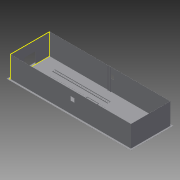
# Autodesk Inventor part: NIST_NRC_Drawing
Saved by Autodesk Inventor 2013 SP2 (Build 170200200, 200)
## iProperties
Created: 2014-01-14
Part Number: NIST_NRC_Drawing
Material: Generic
Document SubType Name: Modeling
Designer: mcgratta
Density: 1 g/cm^3
Author: mcgratta
Autodesk Inventor part; units mm, degrees
ref_plane "YZ Plane" through (0, 0, 0) normal (1, 0, 0) x (0, 1, 0)
ref_plane "XZ Plane" through (0, 0, 0) normal (0, 1, 0) x (-1, 0, 0)
sketch "Sketch1" plane through (0, 0, 0) normal (0, 1, 0) x (-1, 0, 0)
  line L0 (300, 300) -> (-21960, 300)
  line L1 (-21960, 300) -> (-21960, -7340)
  line L2 (-21960, -7340) -> (300, -7340)
  line L3 (300, -7340) -> (300, 300)
  point P0 (0, 0)
  dimension "d0" = 300
  dimension "d1" = 22260
  dimension "d2" = 300
  dimension "d3" = 7640
  constraints: 8 end point, 2 parallel, 1 horizontal, 1 perpendicular
  measures "d0" distance from line of L3 point (0, 0)
  measures "d1" distance between parallel lines of L1 L3
  measures "d2" distance from line of L0 point (0, 0)
  measures "d3" distance between parallel lines of L2 L0
extrude "Extrusion2" add sketch "Sketch1" against normal blind 10
sketch "Sketch4" plane through (0, 0, 0) normal (0, 1, 0) x (1, 0, 0)
  line L0 (0, 0) -> (21700, 0)
  line L1 (21700, 0) -> (21700, 20)
  line L2 (21700, 20) -> (0, 20)
  line L3 (0, 20) -> (0, 0)
  dimension "d28" = 20
  dimension "d30" = 21700
  constraints: 8 end point, 2 parallel, 1 horizontal, 1 perpendicular
  measures "d28" distance between parallel lines of L0 L2
  measures "d30" distance between parallel lines of L1 L3
extrude "Extrusion4" add sketch "Sketch4" along normal blind 3820
sketch "Sketch5" plane through (0, 0, 0) normal (0, 1, 0) x (1, 0, 0)
  line L0 (0, 20) -> (21700, 20) projected
  line L1 (0, 20) -> (20, 20)
  line L2 (20, 20) -> (20, 7060)
  line L3 (20, 7060) -> (0, 7060)
  line L4 (0, 7060) -> (0, 20)
  dimension "d33" = 20
  dimension "d35" = 7040
  constraints: 8 end point, 2 parallel, 1 horizontal, 1 perpendicular
  measures "d33" distance between parallel lines of L2 L4
  measures "d35" distance between parallel lines of L3 L0
extrude "Extrusion5" add sketch "Sketch5" along normal blind 3820
sketch "Sketch6" plane through (0, 0, 0) normal (0, 1, 0) x (1, 0, 0)
  line L0 (0, 7060) -> (21700, 7060)
  line L1 (21700, 7060) -> (21700, 7080)
  line L2 (21700, 7080) -> (0, 7080)
  line L3 (0, 7080) -> (0, 7060)
  dimension "d38" = 20
  dimension "d40" = 21700
  constraints: 8 end point, 2 parallel, 1 horizontal, 1 perpendicular
  measures "d38" distance between parallel lines of L0 L2
  measures "d40" distance between parallel lines of L1 L3
extrude "Extrusion6" add sketch "Sketch6" along normal blind 3820
sketch "Sketch7" plane through (0, 0, 0) normal (0, 1, 0) x (1, 0, 0)
  line L0 (0, 20) -> (21700, 20) projected
  line L1 (21700, 20) -> (21680, 20)
  line L2 (21680, 20) -> (21680, 7060)
  line L3 (21680, 7060) -> (21700, 7060)
  line L4 (21700, 7060) -> (21700, 20)
  point P0 (20, 20)
  dimension "d43" = 20
  dimension "d45" = 7040
  constraints: 8 end point, 2 parallel, 1 horizontal, 1 perpendicular
  measures "d43" distance between parallel lines of L4 L2
  measures "d45" distance between parallel lines of L3 L0
extrude "Extrusion7" add sketch "Sketch7" along normal blind 3820
sketch "Sketch10" plane through (20, 0, -20) normal (1, 0, 0) x (0, 0, -1)
  line L0 (7040, 0) -> (0, 0) projected
  line L1 (7040, 0) -> (7040, 3820) projected
  line L2 (0, 3820) -> (7040, 3820) projected
  line L3 (0, 0) -> (0, 3820) projected
  point P0 (-20, 0)
sketch "Sketch11" plane through (0, 0, 0) normal (-1, 0, 0) x (0, 0, 1)
  line L0 (0, 0) -> (-7080, 0) projected
  line L1 (-7080, 0) -> (-7080, 3820) projected
  line L2 (-4560, 0) -> (-2560, 0)
  line L3 (-2560, 0) -> (-2560, 2000)
  line L4 (-2560, 2000) -> (-4560, 2000)
  line L5 (-4560, 2000) -> (-4560, 0)
  dimension "d73" = 2000
  dimension "d75" = 2000
  dimension "d76" = 2520
  constraints: 8 end point, 2 parallel, 1 horizontal, 1 perpendicular, 1 point on line
  measures "d73" distance between parallel lines of L3 L5
  measures "d75" distance of L2.end L3.end
  measures "d76" distance between parallel lines of L1 L5
extrude "Extrusion10" cut sketch "Sketch11" along normal mid plane 40
sketch "Sketch12" plane through (0, 0, 0) normal (0, 0, 1) x (1, 0, 0)
  line L0 (21700, 0) -> (0, 0) projected
  line L1 (0, 0) -> (0, 3820) projected
  line L2 (10870, 2050) -> (11570, 2050)
  line L3 (11570, 2050) -> (11570, 2750)
  line L4 (11570, 2750) -> (10870, 2750)
  line L5 (10870, 2750) -> (10870, 2050)
  line L6 (10870, 2050) -> (11570, 2750) construction
  line L7 (11570, 2050) -> (10870, 2750) construction
  point P0 (11220, 2400)
  dimension "d79" = 2400
  dimension "d80" = 700
  dimension "d81" = 700
  dimension "d82" = 11220
  constraints: 12 end point, 2 midpoint, 2 parallel, 1 horizontal, 1 perpendicular
  measures "d79" distance from line of L0 point (11220, 2400)
  measures "d80" distance of L2.start L2.end
  measures "d81" distance of L4.end L2.start
  measures "d82" distance from line of L1 point (11220, 2400)
extrude "Extrusion11" cut sketch "Sketch12" along normal mid plane 40
sketch "Sketch13" plane through (21700, 0, -7080) normal (0, 0, -1) x (-1, 0, 0)
  line L0 (21700, 0) -> (0, 0) projected
  line L1 (21700, 0) -> (21700, 3820) projected
  line L2 (10130, 2050) -> (10830, 2050)
  line L3 (10830, 2050) -> (10830, 2750)
  line L4 (10830, 2750) -> (10130, 2750)
  line L5 (10130, 2750) -> (10130, 2050)
  line L6 (10130, 2050) -> (10830, 2750) construction
  line L7 (10830, 2050) -> (10130, 2750) construction
  point P0 (10480, 2400)
  dimension "d85" = 11220
  dimension "d86" = 2400
  dimension "d87" = 700
  dimension "d88" = 700
  constraints: 12 end point, 2 midpoint, 2 parallel, 1 horizontal, 1 perpendicular
  measures "d85" distance from line of L1 point (10480, 2400)
  measures "d86" distance from line of L0 point (10480, 2400)
  measures "d87" distance of L2.start L2.end
  measures "d88" distance of L4.end L2.start
extrude "Extrusion12" cut sketch "Sketch13" against normal blind 40
sketch "Sketch14" plane through (0, 0, 0) normal (0, 1, 0) x (1, 0, 0)
  line L0 (21680, 7060) -> (20, 7060) projected
  line L1 (20, 7060) -> (20, 4560) projected
  line L2 (11850, 3040) -> (9850, 3040)
  line L3 (9850, 3040) -> (9850, 4040)
  line L4 (9850, 4040) -> (11850, 4040)
  line L5 (11850, 4040) -> (11850, 3040)
  line L6 (11850, 3040) -> (9850, 4040) construction
  line L7 (9850, 3040) -> (11850, 4040) construction
  line L8 (9840, 4050) -> (11860, 4050)
  line L9 (11860, 4050) -> (11860, 3030)
  line L10 (11860, 3030) -> (9840, 3030)
  line L11 (9840, 3030) -> (9840, 4050)
  point P0 (10850, 3540)
  point P1 (0, 7060)
  dimension "d91" = 10830
  dimension "d92" = 3520
  dimension "d93" = 2000
  dimension "d94" = 1000
  dimension "d95" = 10
  dimension "d96" = 10
  dimension "d97" = 10
  dimension "d98" = 10
  constraints: 20 end point, 4 parallel, 2 horizontal, 2 midpoint, 2 perpendicular
  measures "d91" distance from line of L1 point (10850, 3540)
  measures "d92" distance from line of L0 point (10850, 3540)
  measures "d93" distance of L2.start L2.end
  measures "d94" distance of L2.end L3.end
  measures "d95" distance between parallel lines of L4 L8
  measures "d96" distance between parallel lines of L3 L11
  measures "d97" distance between parallel lines of L2 L10
  measures "d98" distance between parallel lines of L5 L9
extrude "Extrusion13" add sketch "Sketch14" along normal blind 100
ref_plane "Work Plane1" through (15850, 0, -7060) normal (-1, 0, 0) x (0, 0, 1)
sketch "Sketch16" plane through (15850, 0, -7060) normal (-1, 0, 0) x (0, 0, 1)
  circle A0 centre (4840, 3200) radius 10
  line L0 (-280, 0) -> (7360, 0) projected
  line L1 (7040, 0) -> (7040, 3820) projected
  line L2 (4890, 3210) -> (5340, 3210)
  line L3 (5340, 3210) -> (5340, 3200)
  line L4 (5340, 3200) -> (4890, 3200)
  line L5 (4890, 3200) -> (4890, 3210)
  line L6 (4890, 3210) -> (4900, 3210)
  line L7 (4900, 3210) -> (4900, 3310)
  line L8 (4900, 3310) -> (4890, 3310)
  line L9 (4890, 3310) -> (4890, 3210)
  line L10 (5340, 3210) -> (5330, 3210)
  line L11 (5330, 3210) -> (5330, 3310)
  line L12 (5330, 3310) -> (5340, 3310)
  line L13 (5340, 3310) -> (5340, 3210)
  circle A1 centre (5015, 3220) radius 10
  circle A2 centre (5115, 3220) radius 10
  circle A3 centre (5215, 3220) radius 10
  circle A4 centre (5690, 2700) radius 10
  circle A5 centre (6440, 2200) radius 10
  circle A6 centre (6540, 2200) radius 10
  point P0 (7060, 0)
  dimension "d102" = 3200
  dimension "d103" = 2200
  dimension "d104" = 20
  dimension "d105" = 10
  dimension "d106" = 50
  dimension "d107" = 0
  dimension "d108" = 450
  dimension "d109" = 10
  dimension "d110" = 100
  dimension "d111" = 10
  dimension "d112" = 100
  dimension "d113" = 20
  dimension "d114" = 20
  dimension "d115" = 20
  dimension "d116" = 10
  dimension "d117" = 10
  dimension "d118" = 10
  dimension "d119" = 225
  dimension "d120" = 100
  dimension "d121" = 100
  dimension "d122" = 2700
  dimension "d123" = 1350
  dimension "d124" = 20
  dimension "d125" = 2200
  dimension "d126" = 2200
  dimension "d127" = 600
  dimension "d128" = 500
  dimension "d129" = 20
  dimension "d130" = 20
  constraints: 24 end point, 7 centre point, 6 parallel, 3 horizontal, 3 perpendicular
  measures "d102" distance from line of L0 A0.centre
  measures "d103" distance from line of L1 A0.centre
  measures "d104" diameter of A0
  measures "d105" distance between parallel lines of L4 L2
  measures "d106" horizontal distance of L2.start A0.centre
  measures "d107" distance from line of A0.centre L4
  measures "d108" distance of L3.end L4.end
  measures "d109" distance between parallel lines of L7 L9
  measures "d110" distance of L8.end L2.start
  measures "d111" distance between parallel lines of L13 L11
  measures "d112" vertical distance of L10.end L12.end
  measures "d113" diameter of A1
  measures "d114" diameter of A2
  measures "d115" diameter of A3
  measures "d116" distance from line of L2 A1.centre
  measures "d117" distance from line of L2 A2.centre
  measures "d118" distance from line of L2 A3.centre
  measures "d119" distance from line of L9 A2.centre
  measures "d120" distance of A1.centre A2.centre
  measures "d121" distance of A2.centre A3.centre
  measures "d122" distance from line of L0 A4.centre
  measures "d123" distance from line of L1 A4.centre
  measures "d124" diameter of A4
  measures "d125" distance from line of L0 A5.centre
  measures "d126" distance from line of L0 A6.centre
  measures "d127" distance from line of L1 A5.centre
  measures "d128" distance from line of L1 A6.centre
  measures "d129" diameter of A5
  measures "d130" diameter of A6
extrude "Extrusion14" add sketch "Sketch16" along normal blind 10000
sketch "Sketch17" plane through (0, 0, 0) normal (0, 1, 0) x (1, 0, 0)
  line L0 (21680, 7060) -> (20, 7060) projected
  line L1 (20, 7060) -> (20, 4560) projected
  line L2 (10600, 7010) -> (11050, 7010)
  line L3 (11050, 7010) -> (11050, 7000)
  line L4 (11050, 7000) -> (10600, 7000)
  line L5 (10600, 7000) -> (10600, 7010)
  line L6 (10600, 7000) -> (10610, 7000)
  line L7 (10610, 7000) -> (10610, 6900)
  line L8 (10610, 6900) -> (10600, 6900)
  line L9 (10600, 6900) -> (10600, 7000)
  line L10 (11050, 7000) -> (11040, 7000)
  line L11 (11040, 7000) -> (11040, 6900)
  line L12 (11040, 6900) -> (11050, 6900)
  line L13 (11050, 6900) -> (11050, 7000)
  dimension "d133" = 450
  dimension "d135" = 10
  dimension "d136" = 10
  dimension "d137" = 10
  dimension "d139" = 100
  dimension "d140" = 100
  dimension "d141" = 50
  dimension "d142" = 10580
  constraints: 24 end point, 6 parallel, 3 horizontal, 3 perpendicular
  measures "d133" distance of L2.start L2.end
  measures "d135" distance between parallel lines of L4 L2
  measures "d136" distance between parallel lines of L9 L7
  measures "d137" distance between parallel lines of L13 L11
  measures "d139" distance of L7.end L6.end
  measures "d140" distance of L11.end L10.end
  measures "d141" distance between parallel lines of L2 L0
  measures "d142" distance between parallel lines of L1 L9
extrude "Extrusion15" add sketch "Sketch17" along normal blind 3820
body "Solid1"
